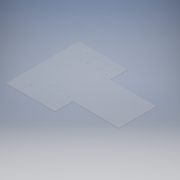
# Autodesk Inventor part: lexan
Saved by Autodesk Inventor 2017 (Build 210142000, 142)
## iProperties
Created: 2020-02-01
Part Number: lexan
Material: PET Plastic
Document SubType Name: Modeling
Designer: S338674153
Density: 1.541 g/cm^3
Appearance: Polycarbonate - Clear
Author: S338674153
Autodesk Inventor part; units mm, degrees
ref_plane "YZ Plane" through (0, 0, 0) normal (1, 0, 0) x (0, 1, 0)
ref_plane "XZ Plane" through (0, 0, 0) normal (0, 1, 0) x (-1, 0, 0)
ref_plane "XY Plane" through (0, 0, 0) normal (0, 0, 1) x (1, 0, 0)
sketch "Sketch1" plane through (0, 0, 0) normal (0, 1, 0) x (-1, 0, 0)
  line L0 (0, 0) -> (266.7, 0)
  line L1 (266.7, -215.9) -> (0, -215.9)
  line L2 (0, -215.9) -> (0, 0)
  line L3 (266.7, 0) -> (266.7, 101.6)
  line L4 (266.7, 101.6) -> (549.275, 101.6)
  line L5 (266.7, -215.9) -> (266.7, -317.5)
  line L6 (266.7, -317.5) -> (549.275, -317.5)
  line L7 (549.275, -317.5) -> (549.275, 101.6)
  dimension "d0" = 266.7
  dimension "d2" = 101.6
  dimension "d3" = 282.575
  dimension "d4" = 101.6
  dimension "d5" = 282.575
  dimension "d6" = 215.9
  constraints: 16 end point, 2 horizontal, 2 vertical, 1 parallel, 1 perpendicular
  measures "d0" distance of L1.start L1.end
  measures "d2" distance of L0.end L3.end
  measures "d3" distance of L3.end L4.end
  measures "d4" distance of L1.start L5.end
  measures "d5" distance of L5.end L6.end
  measures "d6" distance of L1.end L0.start
extrude "Extrusion1" add sketch "Sketch1" along normal blind 2.54
sketch "Sketch3" plane through (0, 0, 0) normal (0, -1, 0) x (1, 0, 0)
  circle A0 centre (-465.7727, -232.3192) radius 2.0915
  circle A1 centre (-465.7727, -283.1146) radius 1.9252
  circle A2 centre (-410.9744, -232.3192) radius 2.0915
  circle A3 centre (-410.9744, -283.1146) radius 1.9252
  circle A4 centre (-356.2402, -232.3192) radius 2.0915
  circle A5 centre (-356.2402, -283.1146) radius 2.0915
  circle A6 centre (-301.3554, -232.3192) radius 2.0915
  circle A7 centre (-301.3554, -283.1146) radius 2.0915
  point P0 (0, 0)
  constraints: 8 centre point
extrude "Extrusion2" cut sketch "Sketch3" against normal up to surface (2.54 mm away)
sketch "Sketch4" plane through (0, 0, 0) normal (0, -1, 0) x (1, 0, 0)
  circle A0 centre (-303.8865, -12.5692) radius 2.0076
  circle A1 centre (-303.8865, 38.2777) radius 1.9477
  circle A2 centre (-358.6531, -12.5692) radius 2.0076
  circle A3 centre (-358.6531, 38.2777) radius 2.0076
  circle A4 centre (-413.6374, -12.5692) radius 2.0076
  circle A5 centre (-413.6374, 38.2777) radius 2.0076
  circle A6 centre (-468.3833, -12.5692) radius 2.0076
  circle A7 centre (-468.3833, 38.2777) radius 2.0076
  point P0 (0, 0)
  constraints: 8 centre point
extrude "Extrusion3" cut sketch "Sketch4" against normal up to surface (2.54 mm away)
body "Solid1"
